GPSmount (Autodesk Fusion 360 design; units mm, degrees)
Autodesk Fusion 360 part; units mm, degrees
sketch "Sketch1" plane through (0, 0, 0) normal (0, 0, 1) x (1, 0, 0)
  line L0 (12.75, -12.75) -> (-12.75, -12.75)
  line L1 (-12.75, -12.75) -> (-12.75, 12.75)
  line L2 (-12.75, 12.75) -> (12.75, 12.75)
  line L3 (12.75, 12.75) -> (12.75, -12.75)
  line L4 (12.75, -12.75) -> (-12.75, 12.75) construction
  line L5 (-12.75, -12.75) -> (12.75, 12.75) construction
  line L6 (-0.75, 12.75) -> (0.75, 12.75)
  line L7 (0.75, 12.75) -> (0.75, 42.75)
  line L8 (0.75, 42.75) -> (-0.75, 42.75)
  line L9 (-0.75, 42.75) -> (-0.75, 12.75)
  dimension "d1" = 25.5
  dimension "d2" = 25.5
  dimension "d3" = 1.5
  dimension "d4" = 30
  dimension "d5" = 0.75
  constraint horizontal L0
  constraint perpendicular L0 L1
  constraint parallel L0 L2
  constraint parallel L1 L3
  constraint coincident L4 origin
  constraint coincident L5 origin
  constraint horizontal L6
  constraint vertical L7
  constraint horizontal L8
  constraint vertical L9
  constraint coincident L2 L6.start
  measures "d1" distance of L1.end L2.end
  measures "d2" distance of L0.end L1.end
  measures "d3" distance of L6.start L6.end
  measures "d4" distance of L6.start L8.end
  measures "d5" horizontal distance of origin L6.start
extrude "Extrude1" add sketch "Sketch1" along normal blind 10 makes body 1
sketch "Sketch2" plane through (0, 0, 10) normal (0, 0, 1) x (-1, 0, 0)
  line L0 (-0.75, -12.75) -> (-0.75, -42.75)
  line L1 (-0.75, -42.75) -> (0.75, -42.75)
  line L2 (0.75, -42.75) -> (0.75, -12.75)
  line L3 (0.75, -12.75) -> (12.75, -12.75)
  line L4 (12.75, -12.75) -> (12.75, 12.75)
  line L5 (12.75, 12.75) -> (-12.75, 12.75)
  line L6 (-12.75, 12.75) -> (-12.75, -12.75)
  line L7 (-12.75, -12.75) -> (-0.75, -12.75)
  line L8 (-15, 15) -> (15, 15)
  line L9 (15, 15) -> (15, -15)
  line L10 (15, -15) -> (-15, -15)
  line L11 (-15, -15) -> (-15, 15)
  line L12 (-15, 15) -> (15, -15) construction
  line L13 (15, 15) -> (-15, -15) construction
  line L14 (-22.5, 15) -> (22.5, 15)
  line L15 (22.5, 15) -> (22.5, -15)
  line L16 (22.5, -15) -> (-22.5, -15)
  line L17 (-22.5, -15) -> (-22.5, 15)
  line L18 (-22.5, 15) -> (22.5, -15) construction
  line L19 (22.5, 15) -> (-22.5, -15) construction
  line L20 (-26.5, 6.65) -> (-18.5, 6.65)
  line L21 (-18.5, 6.65) -> (-18.5, -6.65)
  line L22 (-18.5, -6.65) -> (-26.5, -6.65)
  line L23 (-26.5, -6.65) -> (-26.5, 6.65)
  line L24 (-26.5, 6.65) -> (-18.5, -6.65) construction
  line L25 (-18.5, 6.65) -> (-26.5, -6.65) construction
  line L26 (18.5, 6.65) -> (26.5, 6.65)
  line L27 (26.5, 6.65) -> (26.5, -6.65)
  line L28 (26.5, -6.65) -> (18.5, -6.65)
  line L29 (18.5, -6.65) -> (18.5, 6.65)
  line L30 (18.5, 6.65) -> (26.5, -6.65) construction
  line L31 (26.5, 6.65) -> (18.5, -6.65) construction
  point P0 (-22.5, 0)
  point P1 (22.5, 0)
  dimension "d8" = 30
  dimension "d9" = 30
  dimension "d10" = 45
  dimension "d11" = 30
  dimension "d12" = 8
  dimension "d13" = 13.3
  dimension "d14" = 8
  dimension "d15" = 13.3
  constraint horizontal L8
  constraint perpendicular L8 L9
  constraint parallel L8 L10
  constraint parallel L9 L11
  constraint coincident L12 origin
  constraint coincident L13 origin
  constraint horizontal L14
  constraint perpendicular L14 L15
  constraint parallel L14 L16
  constraint parallel L15 L17
  constraint coincident L18 origin
  constraint coincident L19 origin
  constraint horizontal L20
  constraint perpendicular L20 L21
  constraint parallel L20 L22
  constraint parallel L21 L23
  constraint coincident L24 P0
  constraint coincident L25 P0
  constraint midpoint L17 P0
  constraint horizontal L26
  constraint perpendicular L26 L27
  constraint parallel L26 L28
  constraint parallel L27 L29
  constraint coincident L30 P1
  constraint coincident L31 P1
  constraint midpoint L15 P1
  measures "d8" distance of L9.end L10.end
  measures "d9" distance of L8.end L9.end
  measures "d10" distance of L15.end L16.end
  measures "d11" distance of L14.end L15.end
  measures "d12" distance of L21.end L22.end
  measures "d13" distance of L20.end L21.end
  measures "d14" distance of L27.end L28.end
  measures "d15" distance of L26.end L27.end
extrude "Extrude2" add sketch "Sketch2" against normal blind 10 separate body contours L0 L2 L3 L4 L5 L6 L7 L8 L9 L10 L11 L14 L16 makes body 2
extrude "Extrude3" add sketch "Sketch2" along normal blind 1.5 contours L0 L2 L3 L4 L5 L6 L7 L10 L16 | L0 L2 L3 L4 L5 L6 L7 L8 L9 L10 L11 L14 L16 | L11 L14 L16 L17 L20 L21 L22 | L9 L14 L15 L16 L26 L28 L29 | L17 L20 L21 L22 | L15 L26 L28 L29 bodies 2
extrude "Extrude4" add sketch "Sketch2" against normal blind 0.7 contours L11 L14 L16 L17 L20 L21 L22 | L9 L14 L15 L16 L26 L28 L29 bodies 2
extrude "Extrude5" add sketch "Sketch2" against normal blind 1.5 from surface at -0.7 contours L11 L14 L16 L17 L20 L21 L22 | L9 L14 L15 L16 L26 L28 L29 | L17 L20 L21 L22 | L15 L26 L28 L29 bodies 2
hidden bodies 1
